Autodesk Fusion 360 part; units mm, degrees
(part 2 of 2)
equation "d98 = wood_thickness"
equation "d99 = wood_thickness"
equation "d100 = wood_thickness"
equation "d101 = wood_thickness"
equation "d112 = wood_thickness"
equation "d133 = art_thickness"
